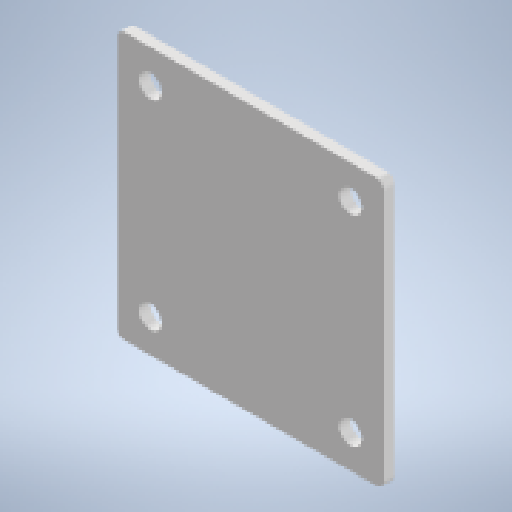
# Autodesk Inventor part: пластина нижняя соед X16
Saved by Autodesk Inventor 2025 (Build 290162010, 162A)
## iProperties
Created: 2024-06-15
Part Number: пластина нижняя соед X16
Material: Generic
Document SubType Name: Sheet Metal
Designer: admin
Density: 1 g/cm^3
Sheet Metal Rule: Default
Appearance: Default
Author: admin
Autodesk Inventor part; units mm, degrees
ref_plane "YZ Plane" through (0, 0, 0) normal (1, 0, 0) x (0, 1, 0)
ref_plane "XZ Plane" through (0, 0, 0) normal (0, 1, 0) x (-1, 0, 0)
ref_plane "XY Plane" through (0, 0, 0) normal (0, 0, 1) x (1, 0, 0)
sketch "Sketch1" plane through (0, 0, 0) normal (0, 1, 0) x (-1, 0, 0)
  line L0 (100, 85) -> (-100, 85)
  line L1 (-100, 85) -> (-100, -85)
  line L2 (-100, -85) -> (100, -85)
  line L3 (100, -85) -> (100, 85)
  point P0 (0, 0)
  point P1 (0, 85)
  point P2 (100, 0)
  dimension "d0" = 200
  dimension "d1" = 170
  measures "d0" distance of L0.start L0.end
  measures "d1" distance of L2.end L0.start
extrude "Plate1" add sketch "Sketch1" along normal blind 8
sketch "Sketch2" plane through (0, 0, 0) normal (0, -1, 0) x (1, 0, 0)
  line L0 (80, 65) -> (80, -65) construction
  line L1 (-100, -85) -> (-100, 85) projected
  line L2 (100, 85) -> (100, -85) projected
  point P0 (0, 0)
  point P1 (80, 0)
  point P2 (-100, 0)
  dimension "d10" = 20
  dimension "d12" = 20
  constraints: 2 end point, 1 coincident, 1 horizontal alignment, 1 midpoint, 1 vertical, 2 other
  measures "d10" distance between parallel lines of L2 L0
  measures "d12" horizontal distance of L0.start L2.start
hole "Hole1" at (80, 0, 65) at (80, 0, -65) direction (0, 1, 0) diameter 17 end through all
fillet "Corner Round1" radius 6 4 edges at (100, 4, 85) (100, 4, -85) (-100, 4, -85) (-100, 4, 85)
mirror "Mirror1" about plane through (0, 0, 0) normal (1, 0, 0) of "Hole1"
equation "\"d12\" = d10"
equation "\"d8\" = Thickness"
equation "\"d2\" = Thickness"
equation "\"BendRadius\" = Thickness"
equation "\"BendReliefWidth\" = Thickness"
equation "\"BendReliefDepth\" = 0.5 * Thickness"
equation "\"CornerReliefSize\" = 4 * Thickness"
equation "\"MinimumRemnant\" = 2 * Thickness"
equation "\"TransitionRadius\" = BendRadius"
equation "\"JacobiRadiusSize\" = BendRadius"
equation "\"GapSize\" = Thickness"
equation "\"Thickness\" = 8"
body "Solid1"
